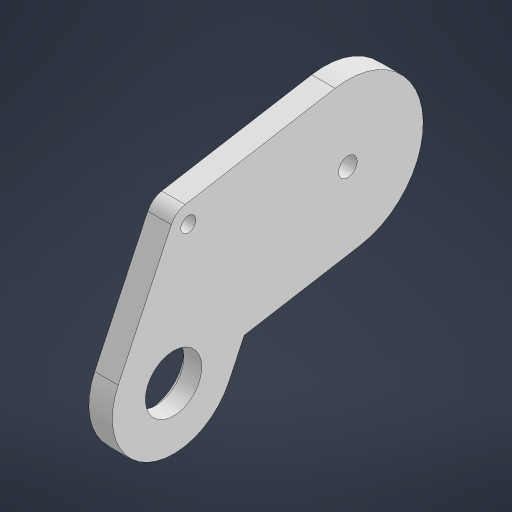
# Autodesk Inventor part: GearCover
Saved by Autodesk Inventor 2024.2 (Build 282272000, 272)
## iProperties
Created: 2023-12-29
Part Number: GearCover
Material: 一般
Document SubType Name: Modeling
Designer: Hanaoka
Density: 1 g/cm^3
Appearance: 既定
Author: Hanaoka
Autodesk Inventor part; units mm, degrees
ref_plane "YZ Plane" through (0, 0, 0) normal (1, 0, 0) x (0, 1, 0)
ref_plane "XZ Plane" through (0, 0, 0) normal (0, 1, 0) x (-1, 0, 0)
ref_plane "XY Plane" through (0, 0, 0) normal (0, 0, 1) x (1, 0, 0)
sketch "スケッチ1" plane through (0, 0, 0) normal (1, 0, 0) x (0, 1, 0)
  circle A0 centre (-10.6702, 18.5052) radius 3.6
  circle A1 centre (-10.6702, 18.5052) radius 3
  arc A2 (-7.8941, 24.3825) -> (-13.4463, 12.6278) centre (-10.6702, 18.5052) ccw
  line L0 (-13.4463, 12.6278) -> (-10, 11)
  line L1 (-10, 11) -> (-7.8852, -1.3502)
  line L2 (7.8852, 1.3502) -> (5.1585, 17.274)
  line L3 (4.0414, 18.7449) -> (-7.8941, 24.3825)
  circle A3 centre (-10.6702, 18.5052) radius 5
  circle A4 centre (-3.4366, 15.0884) radius 3
  arc A5 (5.1585, 17.274) -> (4.0414, 18.7449) centre (3.1872, 16.9365) ccw
  circle A6 centre (3.1872, 16.9365) radius 0.8
  circle A7 centre (3.1872, 16.9365) radius 2 construction
  circle A8 centre (-3.4366, 15.0884) radius 0.75
  line L4 (-10.6702, 18.5052) -> (-3.4366, 15.0884) construction
  arc A9 (-7.8852, -1.3502) -> (7.8852, 1.3502) centre (0, 0) ccw
  circle A10 centre (0, 0) radius 1
  line L5 (-10, 11) -> (-10, 0) construction
  line L6 (-10, 0) -> (0, 0) construction
  point P0 (4.9828, 18.3002)
  dimension "d0" = 6
  dimension "d1" = 7.2
  dimension "d2" = 6.5
  dimension "d7" = 10
  dimension "d8" = 6
  dimension "d9" = 2
  dimension "d10" = 1.6
  dimension "d11" = 4
  dimension "d12" = 1.5
  dimension "d13" = 125
  dimension "d14" = 8
  dimension "d15" = 2
  dimension "d18" = 13.2
  dimension "d19" = 10
  dimension "d20" = 11
  constraints: 14 end point, 11 centre point, 8 coincident, 7 tangent, 6 point on circle, 3 parallel, 2 point on line, 1 perpendicular, 1 vertical
  measures "d0" diameter of A1
  measures "d1" diameter of A0
  measures "d2" radius of A2
  measures "d7" diameter of A3
  measures "d8" diameter of A4
  measures "d9" radius of A5
  measures "d10" diameter of A6
  measures "d11" diameter of A7
  measures "d12" diameter of A8
  measures "d13" angle of L1 L0
  measures "d14" radius of A9
  measures "d15" diameter of A10
  measures "d18" distance of L3.start L3.end
  measures "d19" distance of L5.end L6.end
  measures "d20" distance of L0.end L5.end
extrude "押し出し1" add sketch "スケッチ1" along normal blind 2.5 contours A0 | L3 A5 L2 A9 L1 L0 A2 | A3 | A4 | A8
extrude "押し出し2" cut sketch "スケッチ1" along normal blind 0.6 contours A0
